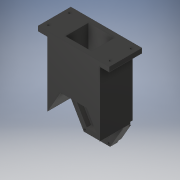
# Autodesk Inventor part: TARM01
Saved by Autodesk Inventor 2017 (Build 210142000, 142)
## iProperties
Created: 2018-10-11
Part Number: TARM01
Material: ABS Plastic
Document SubType Name: Modeling
Designer: Zach
Density: 1.06 g/cm^3
Appearance: Smooth - Black
Author: Zach
Autodesk Inventor part; units mm, degrees
ref_plane "YZ Plane" through (0, 0, 0) normal (1, 0, 0) x (0, 1, 0)
ref_plane "XZ Plane" through (0, 0, 0) normal (0, 1, 0) x (-1, 0, 0)
ref_plane "XY Plane" through (0, 0, 0) normal (0, 0, 1) x (1, 0, 0)
sketch "Sketch5" plane through (0, 0, 0) normal (0, 0, 1) x (1, 0, 0)
  line L0 (56, 0) -> (28, -48.4974)
  line L1 (28, -48.4974) -> (-28, -48.4974)
  line L2 (-28, -48.4974) -> (-56, 0)
  line L3 (-56, 0) -> (-28, 48.4974)
  line L4 (-28, 48.4974) -> (28, 48.4974)
  line L5 (28, 48.4974) -> (56, 0)
  circle A0 centre (0, 30) radius 2.5
  circle A1 centre (-25.9808, 15) radius 2.5
  circle A2 centre (-25.9808, -15) radius 2.5
  circle A3 centre (0, -30) radius 2.5
  circle A4 centre (25.9808, -15) radius 2.5
  circle A5 centre (25.9808, 15) radius 2.5
  point P0 (0, 0)
  point P1 (0, 0)
  dimension "d28" = 112
  dimension "d29" = 5
  dimension "d30" = 30
  dimension "d33" = 360
  constraints: 12 end point, 6 centre point, 1 coincident, 1 horizontal alignment, 1 vertical alignment, 26 other
  measures "d28" distance of L0.start L2.end
  measures "d29" diameter of A0
  measures "d30" distance of point (0, 0) A0.centre
extrude "Extrusion3" add sketch "Sketch5" along normal blind 10
sketch "Sketch6" plane through (0, 0, 10) normal (0, 0, 1) x (1, 0, 0)
  circle A0 centre (25.9808, 15) radius 2.5 construction
  circle A1 centre (25.9808, -15) radius 2.5 construction
  circle A2 centre (0, -30) radius 2.5 construction
  circle A3 centre (-25.9808, -15) radius 2.5 construction
  circle A4 centre (-25.9808, 15) radius 2.5 construction
  circle A5 centre (0, 30) radius 2.5 construction
  line L0 (28, -48.4974) -> (56, 0) projected
  line L1 (56, 0) -> (28, 48.4974) projected
  line L2 (28, 48.4974) -> (-28, 48.4974) projected
  line L3 (-28, 48.4974) -> (-56, 0) projected
  line L4 (-56, 0) -> (-28, -48.4974) projected
  line L5 (-28, -48.4974) -> (28, -48.4974) projected
  line L6 (-44.453, 0) -> (-22.2265, 38.4974)
  line L7 (-22.2265, 38.4974) -> (22.2265, 38.4974)
  line L8 (22.2265, 38.4974) -> (44.453, 0)
  line L9 (44.453, 0) -> (22.2265, -38.4974)
  line L10 (22.2265, -38.4974) -> (-22.2265, -38.4974)
  line L11 (-22.2265, -38.4974) -> (-44.453, 0)
  point P0 (0, 0)
  dimension "d37" = 10
  constraints: 12 end point, 5 other
  measures "d37" distance between parallel lines of L3 L6
extrude "Extrusion4" add sketch "Sketch6" along normal blind 50
sketch "Sketch7" plane through (0, 0, 60) normal (0, 0, 1) x (1, 0, 0)
  line L0 (-22.2265, 38.4974) -> (22.2265, 38.4974) projected
  line L1 (22.2265, 38.4974) -> (44.453, 0) projected
  line L2 (44.453, 0) -> (22.2265, -38.4974) projected
  line L3 (22.2265, -38.4974) -> (-22.2265, -38.4974) projected
  line L4 (-22.2265, -38.4974) -> (-44.453, 0) projected
  line L5 (-44.453, 0) -> (-22.2265, 38.4974) projected
  line L6 (28, -48.4974) -> (56, 0) projected
  line L7 (56, 0) -> (28, 48.4974) projected
  line L8 (28, 48.4974) -> (-28, 48.4974) projected
  line L9 (-28, 48.4974) -> (-56, 0) projected
  line L10 (-56, 0) -> (-28, -48.4974) projected
  line L11 (-28, -48.4974) -> (28, -48.4974) projected
  point P0 (0, 0)
extrude "Extrusion5" add sketch "Sketch7" along normal blind 10 contours L0 L1 L2 L3 L4 L5 | L11 L10 L9 L8 L7 L6
sketch "Sketch8" plane through (-28, 48.4974, 0) normal (0, 1, 0) x (1, 0, 0)
  line L0 (-28, -70) -> (0, -70) projected
  line L1 (-28, -70) -> (84, -70)
  line L2 (84, -70) -> (84, 0)
  line L3 (84, 0) -> (-28, 0)
  line L4 (-28, 0) -> (-28, -70)
  line L5 (0, 0) -> (56, 0) projected
  point P0 (28, 0)
  point P1 (28, 0)
  dimension "d42" = 112
  constraints: 8 end point, 2 midpoint, 2 parallel, 1 horizontal, 1 perpendicular
  measures "d42" distance of L3.end L2.end
extrude "Extrusion6" add sketch "Sketch8" against normal blind 48.4974 and the other way blind 100
sketch "Sketch9" plane through (-28, 148.4974, 0) normal (0, 1, 0) x (1, 0, 0)
  line L0 (-16.453, -60) -> (72.453, -60) projected
  line L1 (72.453, -10) -> (72.453, -60) projected
  line L2 (-16.453, -10) -> (-16.453, -60) projected
  line L3 (50.2265, -10) -> (72.453, -10) projected
  line L4 (72.453, -10) -> (-16.453, -10)
  point P0 (28, 0)
  constraints: 2 end point, 1 collinear
extrude "Extrusion7" cut sketch "Sketch9" against normal blind 100
sketch "Sketch10" plane through (0, 0, 0) normal (0, 0, -1) x (-1, 0, 0)
  circle A0 centre (-25.9808, -15) radius 2.5 projected
  circle A1 centre (-25.9808, -15) radius 2.5 projected
  circle A2 centre (-25.9808, -15) radius 2.5
  circle A3 centre (0, -30) radius 2.5
  circle A4 centre (25.9808, -15) radius 2.5
  circle A5 centre (25.9808, 15) radius 2.5
  circle A6 centre (0, 30) radius 2.5
  circle A7 centre (-25.9808, 15) radius 2.5
  point P0 (0, 0)
  dimension "d52" = 360
  constraints: 6 centre point, 1 coincident, 13 other
extrude "Extrusion8" cut sketch "Sketch10" against normal blind 10
sketch "Sketch12" plane through (0, 0, 70) normal (0, 0, 1) x (1, 0, 0)
  line L0 (56, 0) -> (28, -48.4974) projected
  line L1 (56, 0) -> (28, -48.4974)
  line L2 (28, -48.4974) -> (-28, -48.4974)
  line L3 (-28, -48.4974) -> (-56, 0)
  line L4 (-56, 0) -> (-28, 48.4974)
  line L5 (-28, 48.4974) -> (28, 48.4974)
  line L6 (28, 48.4974) -> (56, 0)
  point P0 (0, 0)
  point P1 (0, 0)
  constraints: 12 end point, 1 coincident, 13 other
extrude "Extrusion9" cut sketch "Sketch12" against normal blind 50
sketch "Sketch13" plane through (0, 0, 10) normal (0, 0, 1) x (1, 0, 0)
  line L0 (22.2265, -38.4974) -> (44.453, 0) projected
  line L1 (22.2265, -38.4974) -> (-22.2265, -38.4974)
  line L2 (-22.2265, -38.4974) -> (-44.453, 0)
  line L3 (-44.453, 0) -> (-22.2265, 38.4974)
  line L4 (-22.2265, 38.4974) -> (22.2265, 38.4974)
  line L5 (22.2265, 38.4974) -> (44.453, 0)
  line L6 (44.453, 0) -> (22.2265, -38.4974)
  point P0 (0, 0)
  point P1 (0, 0)
  constraints: 12 end point, 1 coincident, 13 other
extrude "Extrusion10" cut sketch "Sketch13" along normal blind 10
sketch "Sketch14" plane through (-44.453, 148.4974, 10) normal (0, 0, 1) x (1, 0, 0)
  line L0 (-11.547, -148.4974) -> (16.453, -100) projected
  line L1 (16.453, -100) -> (16.453, -120)
  line L2 (0, -148.4974) -> (22.2265, -110) projected
  line L3 (16.453, -100) -> (72.453, -100) projected
  line L4 (72.453, -100) -> (72.453, -120)
  line L5 (66.6795, -110) -> (88.906, -148.4974) projected
  line L6 (16.453, -120) -> (72.453, -120)
  line L7 (16.453, -100) -> (72.453, -100)
  point P0 (44.453, -148.4974)
  constraints: 8 end point, 2 equal length, 2 point on line, 1 perpendicular, 1 vertical
extrude "Extrusion11" cut sketch "Sketch14" along normal blind 10
sketch "Sketch15" plane through (-28, 148.4974, 0) normal (0, 1, 0) x (1, 0, 0)
  line L0 (-28, -20) -> (-28, -70) projected
  line L1 (-28, -70) -> (-48, -70)
  line L2 (-48, -70) -> (-48, 0)
  line L3 (-48, 0) -> (-28, 0)
  line L4 (-28, 0) -> (-28, -70)
  line L5 (-28, -70) -> (84, -70) projected
  line L6 (84, -70) -> (104, -70)
  line L7 (104, -70) -> (104, 0)
  line L8 (104, 0) -> (84, 0)
  line L9 (84, 0) -> (84, -70)
  circle A0 centre (94, -57.5) radius 2.5
  circle A1 centre (94, -12.5) radius 2.5
  circle A2 centre (-38, -12.5) radius 2.5
  circle A3 centre (-38, -57.5) radius 2.5
  line L10 (94, -57.5) -> (94, -12.5) construction
  line L11 (-38, -12.5) -> (-38, -57.5) construction
  point P0 (28, 0)
  point P1 (-38, -70)
  point P2 (-38, 0)
  point P3 (94, 0)
  point P4 (94, -70)
  point P5 (94, -35)
  point P6 (104, -35)
  dimension "d62" = 20
  dimension "d63" = 20
  dimension "d64" = 5
  dimension "d65" = 5
  dimension "d66" = 5
  dimension "d67" = 5
  dimension "d68" = 45
  constraints: 20 end point, 6 midpoint, 5 parallel, 4 centre point, 4 vertical alignment, 3 horizontal alignment, 2 horizontal, 2 perpendicular, 1 coincident, 1 point on line, 1 vertical
  measures "d62" distance of L7.end L8.end
  measures "d63" distance of L2.end L3.end
  measures "d64" diameter of A0
  measures "d65" diameter of A1
  measures "d66" diameter of A2
  measures "d67" diameter of A3
  measures "d68" distance of L10.start L10.end
extrude "Extrusion12" add sketch "Sketch15" against normal blind 10
sketch "Sketch16" plane through (-28, 48.4974, 0) normal (0, 1, 0) x (1, 0, 0)
  line L0 (0, -20) -> (0, -10) projected
  line L1 (-16.453, -10) -> (0, -10) projected
  line L2 (-16.453, -60) -> (-16.453, -10) projected
  line L3 (0, -60) -> (-16.453, -60) projected
  line L4 (0, -60) -> (0, -20) projected
  line L5 (72.453, -10) -> (72.453, -60) projected
  line L6 (56, -10) -> (56, -20) projected
  line L7 (56, -20) -> (56, -60) projected
  line L8 (72.453, -60) -> (56, -60) projected
  line L9 (72.453, -10) -> (72.453, -60) projected
  line L10 (56, -10) -> (72.453, -10) projected
  point P0 (28, 0)
extrude "Extrusion13" add sketch "Sketch16" along normal blind 100
sketch "Sketch17" plane through (0, 0, 0) normal (0, 0, -1) x (-1, 0, 0)
  circle A0 centre (-51, 0) radius 2.5
  circle A1 centre (-25.5, -44.1673) radius 2.5
  circle A2 centre (25.5, -44.1673) radius 2.5
  circle A3 centre (51, 0) radius 2.5
  circle A4 centre (25.5, 44.1673) radius 2.5
  circle A5 centre (-25.5, 44.1673) radius 2.5
  point P0 (0, 0)
  point P1 (-56, 0)
  dimension "d73" = 5
  dimension "d74" = 5
  dimension "d77" = 360
  constraints: 6 centre point, 1 horizontal alignment, 13 other
  measures "d73" diameter of A0
  measures "d74" distance of point (-56, 0) A0.centre
extrude "Extrusion14" cut sketch "Sketch17" against normal through all
sketch "Sketch18" plane through (0, 0, 0) normal (0, 0, -1) x (-1, 0, 0)
  circle A0 centre (-51, 0) radius 2.5 projected
  circle A1 centre (-51, 0) radius 6.5
  circle A2 centre (-25.5, 44.1673) radius 6.5
  circle A3 centre (25.5, 44.1673) radius 6.5
  circle A4 centre (51, 0) radius 6.5
  circle A5 centre (25.5, -44.1673) radius 6.5
  circle A6 centre (-25.5, -44.1673) radius 6.5
  point P0 (0, 0)
  dimension "d81" = 13
  dimension "d84" = 360
  constraints: 6 centre point, 1 coincident, 13 other
  measures "d81" diameter of A1
extrude "Extrusion15" cut sketch "Sketch18" against normal blind 5 contours A0 | A1 | A2 | A3 | A4 | A5 | A6
sketch "Sketch19" plane through (0, 0, 10) normal (0, 0, 1) x (1, 0, 0)
  circle A0 centre (0, -30) radius 2.5 projected
  circle A1 centre (-25.9808, -15) radius 2.5 projected
  circle A2 centre (-25.9808, 15) radius 2.5 projected
  circle A3 centre (0, 30) radius 2.5 projected
  circle A4 centre (25.9808, 15) radius 2.5 projected
  circle A5 centre (25.9808, -15) radius 2.5 projected
  point P0 (0, 0)
extrude "Extrusion16" add sketch "Sketch19" against normal blind 10
body "Solid2"
